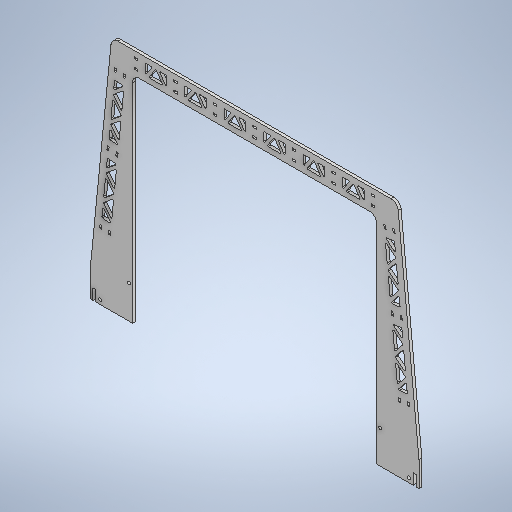
# Autodesk Inventor part: GateBrigeSideLessMaterial
Saved by Autodesk Inventor 2025.1 (Build 291241000, 241)
## iProperties
Created: 2025-03-30
Part Number: GateBrigeSideLessMaterial
Material: Všeobecné
Document SubType Name: Modeling
Designer: 42060
Density: 1 g/cm^3
Appearance: Výchozí
Author: 42060
Autodesk Inventor part; units mm, degrees
ref_plane "YZ Plane" through (0, 0, 0) normal (1, 0, 0) x (0, 1, 0)
ref_plane "XZ Plane" through (0, 0, 0) normal (0, 1, 0) x (-1, 0, 0)
ref_plane "XY Plane" through (0, 0, 0) normal (0, 0, 1) x (1, 0, 0)
sketch "Náčrt1" plane through (0, 0, 0) normal (0, 0, 1) x (1, 0, 0)
  line L0 (0, 0) -> (-160, 0)
  line L1 (-170, -10) -> (-170, -300)
  line L2 (-229, -300) -> (-229, -265.3)
  line L3 (-190.0509, 30) -> (0, 30)
  line L4 (0, 30) -> (0, 0)
  line L5 (-203.7, -249) -> (-170, -249)
  line L6 (-170, -249) -> (-170, -299)
  line L7 (-170, -299) -> (-220, -299)
  line L8 (-220, -299) -> (-220, -265.3)
  line L9 (-220, -265.3) -> (-203.7, -249)
  line L10 (-220, -299) -> (-170, -249) construction
  circle A0 centre (-215, -294) radius 2.1
  circle A1 centre (-175, -254) radius 2.1
  arc A2 (-160, 0) -> (-170, -10) centre (-160, -10) ccw
  line L11 (-200, 21.0077) -> (-229, -265.3)
  arc A3 (-190.0509, 30) -> (-200, 21.0077) centre (-190.0509, 20) ccw
  line L12 (-225, -300) -> (-225, -285)
  line L13 (-225, -285) -> (-221, -285)
  line L14 (-221, -285) -> (-221, -300)
  line L15 (-170, -300) -> (-221, -300)
  line L16 (-225, -300) -> (-229, -300)
  line L17 (0, 0) -> (160, 0)
  line L18 (170, -10) -> (170, -300)
  line L19 (229, -300) -> (229, -265.3)
  line L20 (190.0509, 30) -> (0, 30)
  line L21 (203.7, -249) -> (170, -249)
  line L22 (170, -249) -> (170, -299)
  line L23 (170, -299) -> (220, -299)
  line L24 (220, -299) -> (220, -265.3)
  line L25 (220, -265.3) -> (203.7, -249)
  line L26 (220, -299) -> (170, -249) construction
  circle A4 centre (215, -294) radius 2.1
  circle A5 centre (175, -254) radius 2.1
  arc A6 (170, -10) -> (160, 0) centre (160, -10) ccw
  line L27 (200, 21.0077) -> (229, -265.3)
  arc A7 (200, 21.0077) -> (190.0509, 30) centre (190.0509, 20) ccw
  line L28 (225, -300) -> (225, -285)
  line L29 (225, -285) -> (221, -285)
  line L30 (221, -285) -> (221, -300)
  line L31 (170, -300) -> (221, -300)
  line L32 (225, -300) -> (229, -300)
  line L33 (-36.6095, 9.0611) -> (-28.3278, 21.2788)
  line L34 (-26.6722, 21.2788) -> (-18.3905, 9.0611)
  line L35 (-19.2183, 7.5) -> (-35.7817, 7.5)
  line L36 (-21.6095, 20.9389) -> (-14.3278, 10.1964)
  line L37 (-12.5, 10.7575) -> (-12.5, 21.5)
  line L38 (-13.5, 22.5) -> (-20.7817, 22.5)
  line L39 (-33.3905, 20.9389) -> (-40.6722, 10.1964)
  line L40 (-42.5, 10.7575) -> (-42.5, 21.5)
  line L41 (-41.5, 22.5) -> (-34.2183, 22.5)
  line L42 (-55, 15) -> (0, 15) construction
  arc A8 (-41.5, 22.5) -> (-42.5, 21.5) centre (-41.5, 21.5) ccw
  arc A9 (-33.3905, 20.9389) -> (-34.2183, 22.5) centre (-34.2183, 21.5) ccw
  arc A10 (-42.5, 10.7575) -> (-40.6722, 10.1964) centre (-41.5, 10.7575) ccw
  arc A11 (-36.6095, 9.0611) -> (-35.7817, 7.5) centre (-35.7817, 8.5) ccw
  arc A12 (-19.2183, 7.5) -> (-18.3905, 9.0611) centre (-19.2183, 8.5) ccw
  arc A13 (-26.6722, 21.2788) -> (-28.3278, 21.2788) centre (-27.5, 20.7178) ccw
  arc A14 (-20.7817, 22.5) -> (-21.6095, 20.9389) centre (-20.7817, 21.5) ccw
  arc A15 (-12.5, 21.5) -> (-13.5, 22.5) centre (-13.5, 21.5) ccw
  arc A16 (-14.3278, 10.1964) -> (-12.5, 10.7575) centre (-13.5, 10.7575) ccw
  arc A17 (-81.6722, 21.2788) -> (-83.3278, 21.2788) centre (-82.5, 20.7178) ccw
  line L43 (-91.6095, 9.0611) -> (-83.3278, 21.2788)
  line L44 (-68.5, 22.5) -> (-75.7817, 22.5)
  arc A18 (-67.5, 21.5) -> (-68.5, 22.5) centre (-68.5, 21.5) ccw
  line L45 (-81.6722, 21.2788) -> (-73.3905, 9.0611)
  arc A19 (-74.2183, 7.5) -> (-73.3905, 9.0611) centre (-74.2183, 8.5) ccw
  line L46 (-76.6095, 20.9389) -> (-69.3278, 10.1964)
  line L47 (-74.2183, 7.5) -> (-90.7817, 7.5)
  arc A20 (-69.3278, 10.1964) -> (-67.5, 10.7575) centre (-68.5, 10.7575) ccw
  line L48 (-110, 15) -> (-55, 15) construction
  arc A21 (-96.5, 22.5) -> (-97.5, 21.5) centre (-96.5, 21.5) ccw
  arc A22 (-97.5, 10.7575) -> (-95.6722, 10.1964) centre (-96.5, 10.7575) ccw
  arc A23 (-91.6095, 9.0611) -> (-90.7817, 7.5) centre (-90.7817, 8.5) ccw
  arc A24 (-88.3905, 20.9389) -> (-89.2183, 22.5) centre (-89.2183, 21.5) ccw
  line L49 (-67.5, 10.7575) -> (-67.5, 21.5)
  arc A25 (-75.7817, 22.5) -> (-76.6095, 20.9389) centre (-75.7817, 21.5) ccw
  line L50 (-96.5, 22.5) -> (-89.2183, 22.5)
  line L51 (-88.3905, 20.9389) -> (-95.6722, 10.1964)
  line L52 (-97.5, 10.7575) -> (-97.5, 21.5)
  arc A26 (-136.6722, 21.2788) -> (-138.3278, 21.2788) centre (-137.5, 20.7178) ccw
  line L53 (-146.6095, 9.0611) -> (-138.3278, 21.2788)
  line L54 (-123.5, 22.5) -> (-130.7817, 22.5)
  arc A27 (-122.5, 21.5) -> (-123.5, 22.5) centre (-123.5, 21.5) ccw
  line L55 (-136.6722, 21.2788) -> (-128.3905, 9.0611)
  arc A28 (-129.2183, 7.5) -> (-128.3905, 9.0611) centre (-129.2183, 8.5) ccw
  line L56 (-131.6095, 20.9389) -> (-124.3278, 10.1964)
  line L57 (-129.2183, 7.5) -> (-145.7817, 7.5)
  arc A29 (-124.3278, 10.1964) -> (-122.5, 10.7575) centre (-123.5, 10.7575) ccw
  line L58 (-165, 15) -> (-110, 15) construction
  arc A30 (-151.5, 22.5) -> (-152.5, 21.5) centre (-151.5, 21.5) ccw
  arc A31 (-152.5, 10.7575) -> (-150.6722, 10.1964) centre (-151.5, 10.7575) ccw
  arc A32 (-146.6095, 9.0611) -> (-145.7817, 7.5) centre (-145.7817, 8.5) ccw
  arc A33 (-143.3905, 20.9389) -> (-144.2183, 22.5) centre (-144.2183, 21.5) ccw
  line L59 (-122.5, 10.7575) -> (-122.5, 21.5)
  arc A34 (-130.7817, 22.5) -> (-131.6095, 20.9389) centre (-130.7817, 21.5) ccw
  line L60 (-151.5, 22.5) -> (-144.2183, 22.5)
  line L61 (-143.3905, 20.9389) -> (-150.6722, 10.1964)
  line L62 (-152.5, 10.7575) -> (-152.5, 21.5)
  line L63 (-193.9606, -18.9513) -> (-184.0822, -19.9519)
  line L64 (-183.5507, -21.7216) -> (-194.4297, -30.5994)
  line L65 (-196.0568, -29.7239) -> (-195.0562, -19.8455)
  line L66 (-182.4936, -28.2252) -> (-184.6963, -49.9718)
  line L67 (-186.466, -50.5033) -> (-196.2379, -38.5286)
  line L68 (-196.0954, -37.1216) -> (-184.1208, -27.3497)
  line L69 (-195.9139, -45.2524) -> (-186.1419, -57.227)
  line L70 (-186.2844, -58.634) -> (-198.2591, -68.406)
  line L71 (-199.8862, -67.5304) -> (-197.6835, -45.7838)
  line L72 (-187.9502, -65.1562) -> (-199.9248, -74.9282)
  line L73 (-200.0673, -76.3352) -> (-190.2954, -88.3098)
  line L74 (-188.5257, -87.7783) -> (-186.323, -66.0318)
  line L75 (-199.7433, -83.0589) -> (-190.8655, -93.9379)
  line L76 (-191.741, -95.565) -> (-201.6194, -94.5645)
  line L77 (-202.5135, -93.4688) -> (-201.5129, -83.5904)
  line L78 (-189.0214, -19.4516) -> (-188.064, -10) construction
  arc A35 (-193.9606, -18.9513) -> (-195.0562, -19.8455) centre (-194.0613, -19.9463) ccw
  arc A36 (-183.5507, -21.7216) -> (-184.0822, -19.9519) centre (-184.1829, -20.9468) ccw
  arc A37 (-196.0568, -29.7239) -> (-194.4297, -30.5994) centre (-195.0619, -29.8246) ccw
  arc A38 (-196.0954, -37.1216) -> (-196.2379, -38.5286) centre (-195.4632, -37.8964) ccw
  arc A39 (-186.466, -50.5033) -> (-184.6963, -49.9718) centre (-185.6912, -49.871) ccw
  arc A40 (-182.4936, -28.2252) -> (-184.1208, -27.3497) centre (-183.4885, -28.1244) ccw
  arc A41 (-195.9139, -45.2524) -> (-197.6835, -45.7838) centre (-196.6886, -45.8846) ccw
  arc A42 (-186.2844, -58.634) -> (-186.1419, -57.227) centre (-186.9167, -57.8593) ccw
  arc A43 (-199.8862, -67.5304) -> (-198.2591, -68.406) centre (-198.8913, -67.6312) ccw
  arc A44 (-199.9248, -74.9282) -> (-200.0673, -76.3352) centre (-199.2926, -75.7029) ccw
  arc A45 (-190.2954, -88.3098) -> (-188.5257, -87.7783) centre (-189.5206, -87.6776) ccw
  arc A46 (-186.323, -66.0318) -> (-187.9502, -65.1562) centre (-187.3179, -65.931) ccw
  arc A47 (-199.7433, -83.0589) -> (-201.5129, -83.5904) centre (-200.518, -83.6912) ccw
  arc A48 (-202.5135, -93.4688) -> (-201.6194, -94.5645) centre (-201.5186, -93.5696) ccw
  arc A49 (-191.741, -95.565) -> (-190.8655, -93.9379) centre (-191.6402, -94.5701) ccw
  arc A50 (-212.5909, -192.9597) -> (-211.6968, -194.0554) centre (-211.596, -193.0605) ccw
  line L79 (-201.8184, -195.056) -> (-211.6968, -194.0554)
  arc A51 (-201.8184, -195.056) -> (-200.9429, -193.4288) centre (-201.7176, -194.0611) ccw
  arc A52 (-200.3728, -187.8008) -> (-198.6031, -187.2693) centre (-199.598, -187.1685) ccw
  line L80 (-209.8207, -182.5498) -> (-200.9429, -193.4288)
  line L81 (-212.5909, -192.9597) -> (-211.5903, -183.0813)
  arc A53 (-209.8207, -182.5498) -> (-211.5903, -183.0813) centre (-210.5954, -183.1821) ccw
  line L82 (-198.0276, -164.6471) -> (-210.0022, -174.4191)
  line L83 (-210.1447, -175.8261) -> (-200.3728, -187.8008)
  line L84 (-198.6031, -187.2693) -> (-196.4004, -165.5227)
  arc A54 (-210.0022, -174.4191) -> (-210.1447, -175.8261) centre (-209.37, -175.1939) ccw
  arc A55 (-209.9636, -167.0214) -> (-208.3365, -167.8969) centre (-208.9687, -167.1221) ccw
  arc A56 (-196.4004, -165.5227) -> (-198.0276, -164.6471) centre (-197.3953, -165.4219) ccw
  line L85 (-205.9913, -144.7433) -> (-196.2193, -156.7179)
  arc A57 (-196.3618, -158.125) -> (-196.2193, -156.7179) centre (-196.9941, -157.3502) ccw
  line L86 (-209.9636, -167.0214) -> (-207.7609, -145.2748)
  line L87 (-196.3618, -158.125) -> (-208.3365, -167.8969)
  arc A58 (-196.5434, -149.9942) -> (-194.7737, -149.4627) centre (-195.7686, -149.362) ccw
  arc A59 (-205.9913, -144.7433) -> (-207.7609, -145.2748) centre (-206.766, -145.3755) ccw
  line L88 (-196.5434, -149.9942) -> (-206.3153, -138.0196)
  arc A60 (-206.1728, -136.6125) -> (-206.3153, -138.0196) centre (-205.5406, -137.3873) ccw
  arc A61 (-206.1342, -129.2148) -> (-204.5071, -130.0903) centre (-205.1393, -129.3156) ccw
  line L89 (-192.571, -127.7161) -> (-194.7737, -149.4627)
  line L90 (-206.1728, -136.6125) -> (-194.1982, -126.8406)
  arc A62 (-192.571, -127.7161) -> (-194.1982, -126.8406) centre (-193.5659, -127.6154) ccw
  arc A63 (-193.6281, -121.2125) -> (-194.1596, -119.4429) centre (-194.2603, -120.4378) ccw
  line L91 (-199.0988, -118.9426) -> (-198.1414, -109.4909) construction
  line L92 (-204.038, -118.4423) -> (-194.1596, -119.4429)
  arc A64 (-204.038, -118.4423) -> (-205.1336, -119.3364) centre (-204.1387, -119.4372) ccw
  line L93 (-193.6281, -121.2125) -> (-204.5071, -130.0903)
  line L94 (-206.1342, -129.2148) -> (-205.1336, -119.3364)
  line L95 (36.6095, 9.0611) -> (28.3278, 21.2788)
  line L96 (26.6722, 21.2788) -> (18.3905, 9.0611)
  line L97 (19.2183, 7.5) -> (35.7817, 7.5)
  line L98 (21.6095, 20.9389) -> (14.3278, 10.1964)
  line L99 (12.5, 10.7575) -> (12.5, 21.5)
  line L100 (13.5, 22.5) -> (20.7817, 22.5)
  line L101 (33.3905, 20.9389) -> (40.6722, 10.1964)
  line L102 (42.5, 10.7575) -> (42.5, 21.5)
  line L103 (41.5, 22.5) -> (34.2183, 22.5)
  line L104 (55, 15) -> (0, 15) construction
  arc A65 (42.5, 21.5) -> (41.5, 22.5) centre (41.5, 21.5) ccw
  arc A66 (34.2183, 22.5) -> (33.3905, 20.9389) centre (34.2183, 21.5) ccw
  arc A67 (40.6722, 10.1964) -> (42.5, 10.7575) centre (41.5, 10.7575) ccw
  arc A68 (35.7817, 7.5) -> (36.6095, 9.0611) centre (35.7817, 8.5) ccw
  arc A69 (18.3905, 9.0611) -> (19.2183, 7.5) centre (19.2183, 8.5) ccw
  arc A70 (28.3278, 21.2788) -> (26.6722, 21.2788) centre (27.5, 20.7178) ccw
  arc A71 (21.6095, 20.9389) -> (20.7817, 22.5) centre (20.7817, 21.5) ccw
  arc A72 (13.5, 22.5) -> (12.5, 21.5) centre (13.5, 21.5) ccw
  arc A73 (12.5, 10.7575) -> (14.3278, 10.1964) centre (13.5, 10.7575) ccw
  line L105 (67.5, 10.7575) -> (67.5, 21.5)
  line L106 (96.5, 22.5) -> (89.2183, 22.5)
  arc A74 (97.5, 21.5) -> (96.5, 22.5) centre (96.5, 21.5) ccw
  line L107 (97.5, 10.7575) -> (97.5, 21.5)
  arc A75 (95.6722, 10.1964) -> (97.5, 10.7575) centre (96.5, 10.7575) ccw
  arc A76 (67.5, 10.7575) -> (69.3278, 10.1964) centre (68.5, 10.7575) ccw
  arc A77 (68.5, 22.5) -> (67.5, 21.5) centre (68.5, 21.5) ccw
  arc A78 (89.2183, 22.5) -> (88.3905, 20.9389) centre (89.2183, 21.5) ccw
  arc A79 (83.3278, 21.2788) -> (81.6722, 21.2788) centre (82.5, 20.7178) ccw
  line L108 (88.3905, 20.9389) -> (95.6722, 10.1964)
  line L109 (91.6095, 9.0611) -> (83.3278, 21.2788)
  arc A80 (76.6095, 20.9389) -> (75.7817, 22.5) centre (75.7817, 21.5) ccw
  arc A81 (90.7817, 7.5) -> (91.6095, 9.0611) centre (90.7817, 8.5) ccw
  line L110 (110, 15) -> (55, 15) construction
  line L111 (68.5, 22.5) -> (75.7817, 22.5)
  line L112 (76.6095, 20.9389) -> (69.3278, 10.1964)
  line L113 (81.6722, 21.2788) -> (73.3905, 9.0611)
  arc A82 (73.3905, 9.0611) -> (74.2183, 7.5) centre (74.2183, 8.5) ccw
  line L114 (74.2183, 7.5) -> (90.7817, 7.5)
  line L115 (122.5, 10.7575) -> (122.5, 21.5)
  line L116 (151.5, 22.5) -> (144.2183, 22.5)
  arc A83 (152.5, 21.5) -> (151.5, 22.5) centre (151.5, 21.5) ccw
  line L117 (152.5, 10.7575) -> (152.5, 21.5)
  arc A84 (150.6722, 10.1964) -> (152.5, 10.7575) centre (151.5, 10.7575) ccw
  arc A85 (122.5, 10.7575) -> (124.3278, 10.1964) centre (123.5, 10.7575) ccw
  arc A86 (123.5, 22.5) -> (122.5, 21.5) centre (123.5, 21.5) ccw
  arc A87 (144.2183, 22.5) -> (143.3905, 20.9389) centre (144.2183, 21.5) ccw
  arc A88 (138.3278, 21.2788) -> (136.6722, 21.2788) centre (137.5, 20.7178) ccw
  line L118 (143.3905, 20.9389) -> (150.6722, 10.1964)
  line L119 (146.6095, 9.0611) -> (138.3278, 21.2788)
  arc A89 (131.6095, 20.9389) -> (130.7817, 22.5) centre (130.7817, 21.5) ccw
  arc A90 (145.7817, 7.5) -> (146.6095, 9.0611) centre (145.7817, 8.5) ccw
  line L120 (165, 15) -> (110, 15) construction
  line L121 (123.5, 22.5) -> (130.7817, 22.5)
  line L122 (131.6095, 20.9389) -> (124.3278, 10.1964)
  line L123 (136.6722, 21.2788) -> (128.3905, 9.0611)
  arc A91 (128.3905, 9.0611) -> (129.2183, 7.5) centre (129.2183, 8.5) ccw
  line L124 (129.2183, 7.5) -> (145.7817, 7.5)
  line L125 (193.9606, -18.9513) -> (184.0822, -19.9519)
  line L126 (183.5507, -21.7216) -> (194.4297, -30.5994)
  line L127 (196.0568, -29.7239) -> (195.0562, -19.8455)
  line L128 (182.4936, -28.2252) -> (184.6963, -49.9718)
  line L129 (186.466, -50.5033) -> (196.2379, -38.5286)
  line L130 (196.0954, -37.1216) -> (184.1208, -27.3497)
  line L131 (195.9139, -45.2524) -> (186.1419, -57.227)
  line L132 (186.2844, -58.634) -> (198.2591, -68.406)
  line L133 (199.8862, -67.5304) -> (197.6835, -45.7838)
  line L134 (187.9502, -65.1562) -> (199.9248, -74.9282)
  line L135 (200.0673, -76.3352) -> (190.2954, -88.3098)
  line L136 (188.5257, -87.7783) -> (186.323, -66.0318)
  line L137 (199.7433, -83.0589) -> (190.8655, -93.9379)
  line L138 (191.741, -95.565) -> (201.6194, -94.5645)
  line L139 (202.5135, -93.4688) -> (201.5129, -83.5904)
  arc A92 (195.0562, -19.8455) -> (193.9606, -18.9513) centre (194.0613, -19.9463) ccw
  arc A93 (184.0822, -19.9519) -> (183.5507, -21.7216) centre (184.1829, -20.9468) ccw
  arc A94 (194.4297, -30.5994) -> (196.0568, -29.7239) centre (195.0619, -29.8246) ccw
  arc A95 (196.2379, -38.5286) -> (196.0954, -37.1216) centre (195.4632, -37.8964) ccw
  arc A96 (184.6963, -49.9718) -> (186.466, -50.5033) centre (185.6912, -49.871) ccw
  arc A97 (184.1208, -27.3497) -> (182.4936, -28.2252) centre (183.4885, -28.1244) ccw
  arc A98 (197.6835, -45.7838) -> (195.9139, -45.2524) centre (196.6886, -45.8846) ccw
  arc A99 (186.1419, -57.227) -> (186.2844, -58.634) centre (186.9167, -57.8593) ccw
  arc A100 (198.2591, -68.406) -> (199.8862, -67.5304) centre (198.8913, -67.6312) ccw
  arc A101 (200.0673, -76.3352) -> (199.9248, -74.9282) centre (199.2926, -75.7029) ccw
  arc A102 (188.5257, -87.7783) -> (190.2954, -88.3098) centre (189.5206, -87.6776) ccw
  arc A103 (187.9502, -65.1562) -> (186.323, -66.0318) centre (187.3179, -65.931) ccw
  arc A104 (201.5129, -83.5904) -> (199.7433, -83.0589) centre (200.518, -83.6912) ccw
  arc A105 (201.6194, -94.5645) -> (202.5135, -93.4688) centre (201.5186, -93.5696) ccw
  arc A106 (190.8655, -93.9379) -> (191.741, -95.565) centre (191.6402, -94.5701) ccw
  arc A107 (194.1596, -119.4429) -> (193.6281, -121.2125) centre (194.2603, -120.4378) ccw
  arc A108 (194.1982, -126.8406) -> (192.571, -127.7161) centre (193.5659, -127.6154) ccw
  line L140 (204.038, -118.4423) -> (194.1596, -119.4429)
  line L141 (193.6281, -121.2125) -> (204.5071, -130.0903)
  line L142 (206.1342, -129.2148) -> (205.1336, -119.3364)
  line L143 (206.1728, -136.6125) -> (194.1982, -126.8406)
  arc A109 (205.1336, -119.3364) -> (204.038, -118.4423) centre (204.1387, -119.4372) ccw
  arc A110 (204.5071, -130.0903) -> (206.1342, -129.2148) centre (205.1393, -129.3156) ccw
  line L144 (192.571, -127.7161) -> (194.7737, -149.4627)
  arc A111 (207.7609, -145.2748) -> (205.9913, -144.7433) centre (206.766, -145.3755) ccw
  line L145 (196.5434, -149.9942) -> (206.3153, -138.0196)
  arc A112 (206.3153, -138.0196) -> (206.1728, -136.6125) centre (205.5406, -137.3873) ccw
  arc A113 (194.7737, -149.4627) -> (196.5434, -149.9942) centre (195.7686, -149.362) ccw
  line L146 (205.9913, -144.7433) -> (196.2193, -156.7179)
  arc A114 (196.2193, -156.7179) -> (196.3618, -158.125) centre (196.9941, -157.3502) ccw
  arc A115 (198.0276, -164.6471) -> (196.4004, -165.5227) centre (197.3953, -165.4219) ccw
  line L147 (196.3618, -158.125) -> (208.3365, -167.8969)
  arc A116 (208.3365, -167.8969) -> (209.9636, -167.0214) centre (208.9687, -167.1221) ccw
  line L148 (209.9636, -167.0214) -> (207.7609, -145.2748)
  arc A117 (200.9429, -193.4288) -> (201.8184, -195.056) centre (201.7176, -194.0611) ccw
  arc A118 (211.6968, -194.0554) -> (212.5909, -192.9597) centre (211.596, -193.0605) ccw
  arc A119 (198.6031, -187.2693) -> (200.3728, -187.8008) centre (199.598, -187.1685) ccw
  line L149 (212.5909, -192.9597) -> (211.5903, -183.0813)
  line L150 (209.8207, -182.5498) -> (200.9429, -193.4288)
  arc A120 (211.5903, -183.0813) -> (209.8207, -182.5498) centre (210.5954, -183.1821) ccw
  line L151 (210.1447, -175.8261) -> (200.3728, -187.8008)
  arc A121 (210.1447, -175.8261) -> (210.0022, -174.4191) centre (209.37, -175.1939) ccw
  line L152 (198.6031, -187.2693) -> (196.4004, -165.5227)
  line L153 (198.0276, -164.6471) -> (210.0022, -174.4191)
  line L154 (201.8184, -195.056) -> (211.6968, -194.0554)
  line L155 (-2.5, 10) -> (2.5, 10)
  line L156 (2.5, 10) -> (2.5, 7.5)
  line L157 (2.5, 7.5) -> (-2.5, 7.5)
  line L158 (-2.5, 7.5) -> (-2.5, 10)
  line L159 (-2.5, 22.5) -> (2.5, 22.5)
  line L160 (2.5, 22.5) -> (2.5, 20)
  line L161 (2.5, 20) -> (-2.5, 20)
  line L162 (-2.5, 20) -> (-2.5, 22.5)
  line L163 (0, 20) -> (0, 10) construction
  line L164 (-42.5, 10.7575) -> (-42.5, 7.5) construction
  line L165 (-42.5, 7.5) -> (-40.6722, 10.1964) construction
  line L166 (-27.5, 22.5) -> (-27.5, 7.5) construction
  line L167 (-52.5, 10) -> (-52.5, 7.5)
  line L168 (-57.5, 10) -> (-52.5, 10)
  line L169 (-52.5, 7.5) -> (-57.5, 7.5)
  line L170 (-57.5, 7.5) -> (-57.5, 10)
  line L171 (-57.5, 22.5) -> (-52.5, 22.5)
  line L172 (-52.5, 20) -> (-57.5, 20)
  line L173 (-57.5, 20) -> (-57.5, 22.5)
  line L174 (-52.5, 22.5) -> (-52.5, 20)
  line L175 (-107.5, 10) -> (-107.5, 7.5)
  line L176 (-112.5, 10) -> (-107.5, 10)
  line L177 (-107.5, 7.5) -> (-112.5, 7.5)
  line L178 (-112.5, 7.5) -> (-112.5, 10)
  line L179 (-112.5, 22.5) -> (-107.5, 22.5)
  line L180 (-107.5, 20) -> (-112.5, 20)
  line L181 (-112.5, 20) -> (-112.5, 22.5)
  line L182 (-107.5, 22.5) -> (-107.5, 20)
  line L183 (-162.5, 10) -> (-162.5, 7.5)
  line L184 (-167.5, 10) -> (-162.5, 10)
  line L185 (-162.5, 7.5) -> (-167.5, 7.5)
  line L186 (-167.5, 7.5) -> (-167.5, 10)
  line L187 (-167.5, 22.5) -> (-162.5, 22.5)
  line L188 (-162.5, 20) -> (-167.5, 20)
  line L189 (-167.5, 20) -> (-167.5, 22.5)
  line L190 (-162.5, 22.5) -> (-162.5, 20)
  line L191 (52.5, 20) -> (52.5, 22.5)
  line L192 (57.5, 20) -> (52.5, 20)
  line L193 (57.5, 22.5) -> (57.5, 20)
  line L194 (52.5, 22.5) -> (57.5, 22.5)
  line L195 (57.5, 10) -> (57.5, 7.5)
  line L196 (52.5, 10) -> (57.5, 10)
  line L197 (57.5, 7.5) -> (52.5, 7.5)
  line L198 (52.5, 7.5) -> (52.5, 10)
  line L199 (107.5, 20) -> (107.5, 22.5)
  line L200 (112.5, 20) -> (107.5, 20)
  line L201 (112.5, 22.5) -> (112.5, 20)
  line L202 (107.5, 22.5) -> (112.5, 22.5)
  line L203 (112.5, 10) -> (112.5, 7.5)
  line L204 (107.5, 10) -> (112.5, 10)
  line L205 (112.5, 7.5) -> (107.5, 7.5)
  line L206 (107.5, 7.5) -> (107.5, 10)
  line L207 (162.5, 20) -> (162.5, 22.5)
  line L208 (167.5, 20) -> (162.5, 20)
  line L209 (167.5, 22.5) -> (167.5, 20)
  line L210 (162.5, 22.5) -> (167.5, 22.5)
  line L211 (167.5, 10) -> (167.5, 7.5)
  line L212 (162.5, 10) -> (167.5, 10)
  line L213 (167.5, 7.5) -> (162.5, 7.5)
  line L214 (162.5, 7.5) -> (162.5, 10)
  line L215 (-195.022, -4.2696) -> (-192.5347, -4.5216)
  line L216 (-192.5347, -4.5216) -> (-193.0386, -9.4961)
  line L217 (-193.0386, -9.4961) -> (-195.5258, -9.2442)
  line L218 (-195.5258, -9.2442) -> (-195.022, -4.2696)
  line L219 (-182.5856, -5.5293) -> (-180.0983, -5.7813)
  line L220 (-180.0983, -5.7813) -> (-180.6022, -10.7558)
  line L221 (-180.6022, -10.7558) -> (-183.0895, -10.5039)
  line L222 (-183.0895, -10.5039) -> (-182.5856, -5.5293)
  line L223 (-193.0386, -9.4961) -> (-183.0895, -10.5039) construction
  line L224 (-205.6032, -108.7351) -> (-205.0994, -103.7606)
  line L225 (-202.6121, -104.0125) -> (-203.116, -108.9871)
  line L226 (-203.116, -108.9871) -> (-205.6032, -108.7351)
  line L227 (-205.0994, -103.7606) -> (-202.6121, -104.0125)
  line L228 (-193.1669, -109.9948) -> (-192.663, -105.0203)
  line L229 (-190.6796, -110.2467) -> (-193.1669, -109.9948)
  line L230 (-190.1757, -105.2722) -> (-190.6796, -110.2467)
  line L231 (-192.663, -105.0203) -> (-190.1757, -105.2722)
  line L232 (-203.116, -108.9871) -> (-193.1669, -109.9948) construction
  line L233 (-202.6121, -104.0125) -> (-192.663, -105.0203) construction
  line L234 (-197.6375, -104.5164) -> (-196.6802, -95.0647) construction
  line L235 (-215.6806, -208.2261) -> (-215.1768, -203.2515)
  line L236 (-212.6895, -203.5035) -> (-213.1934, -208.478)
  line L237 (-213.1934, -208.478) -> (-215.6806, -208.2261)
  line L238 (-215.1768, -203.2515) -> (-212.6895, -203.5035)
  line L239 (-203.2443, -209.4857) -> (-202.7404, -204.5112)
  line L240 (-200.757, -209.7377) -> (-203.2443, -209.4857)
  line L241 (-200.2531, -204.7631) -> (-200.757, -209.7377)
  line L242 (-202.7404, -204.5112) -> (-200.2531, -204.7631)
  line L243 (-213.1934, -208.478) -> (-203.2443, -209.4857) construction
  line L244 (195.022, -4.2696) -> (192.5347, -4.5216)
  line L245 (192.5347, -4.5216) -> (193.0386, -9.4961)
  line L246 (193.0386, -9.4961) -> (195.5258, -9.2442)
  line L247 (195.5258, -9.2442) -> (195.022, -4.2696)
  line L248 (182.5856, -5.5293) -> (180.0983, -5.7813)
  line L249 (180.0983, -5.7813) -> (180.6022, -10.7558)
  line L250 (180.6022, -10.7558) -> (183.0895, -10.5039)
  line L251 (183.0895, -10.5039) -> (182.5856, -5.5293)
  line L252 (205.6032, -108.7351) -> (205.0994, -103.7606)
  line L253 (202.6121, -104.0125) -> (203.116, -108.9871)
  line L254 (203.116, -108.9871) -> (205.6032, -108.7351)
  line L255 (205.0994, -103.7606) -> (202.6121, -104.0125)
  line L256 (193.1669, -109.9948) -> (192.663, -105.0203)
  line L257 (190.6796, -110.2467) -> (193.1669, -109.9948)
  line L258 (190.1757, -105.2722) -> (190.6796, -110.2467)
  line L259 (192.663, -105.0203) -> (190.1757, -105.2722)
  line L260 (215.6806, -208.2261) -> (215.1768, -203.2515)
  line L261 (212.6895, -203.5035) -> (213.1934, -208.478)
  line L262 (213.1934, -208.478) -> (215.6806, -208.2261)
  line L263 (215.1768, -203.2515) -> (212.6895, -203.5035)
  line L264 (203.2443, -209.4857) -> (202.7404, -204.5112)
  line L265 (200.757, -209.7377) -> (203.2443, -209.4857)
  line L266 (200.2531, -204.7631) -> (200.757, -209.7377)
  line L267 (202.7404, -204.5112) -> (200.2531, -204.7631)
  point P0 (-12.5, 7.5)
  point P1 (-32.3323, 22.5)
  point P2 (-42.5, 22.5)
  point P3 (-27.5, 15)
  point P4 (-12.5, 16.1288)
  point P5 (-82.5, 22.5)
  point P6 (-82.5, 15)
  point P7 (-82.5, 7.5)
  point P8 (-87.3323, 22.5)
  point P9 (-97.5, 22.5)
  point P10 (-67.5, 7.5)
  point P11 (-67.5, 16.1288)
  point P12 (-137.5, 22.5)
  point P13 (-137.5, 15)
  point P14 (-137.5, 7.5)
  point P15 (-142.3323, 22.5)
  point P16 (-152.5, 22.5)
  point P17 (-122.5, 7.5)
  point P18 (-122.5, 16.1288)
  point P19 (-194.9555, -18.8506)
  point P20 (-181.6802, -20.1952)
  point P21 (-196.3001, -32.1258)
  point P22 (-182.2503, -25.8233)
  point P23 (-184.9396, -52.3737)
  point P24 (-196.8702, -37.7539)
  point P25 (-197.4402, -43.3819)
  point P26 (-185.5097, -58.0018)
  point P27 (-200.1295, -69.9324)
  point P28 (-186.0797, -63.6298)
  point P29 (-200.6996, -75.5604)
  point P30 (-188.769, -90.1803)
  point P31 (-201.2696, -81.1885)
  point P32 (-189.3391, -95.8083)
  point P33 (-202.6143, -94.4637)
  point P34 (-212.6917, -193.9546)
  point P35 (-199.4165, -195.2993)
  point P36 (-198.8464, -189.6712)
  point P37 (-211.347, -180.6794)
  point P38 (-210.777, -175.0513)
  point P39 (-210.2069, -169.4233)
  point P40 (-196.1571, -163.1208)
  point P41 (-195.5871, -157.4927)
  point P42 (-195.017, -151.8647)
  point P43 (-207.5176, -142.8728)
  point P44 (-206.9476, -137.2448)
  point P45 (-206.3775, -131.6167)
  point P46 (-192.3277, -125.3142)
  point P47 (-191.7576, -119.6862)
  point P48 (-205.0329, -118.3415)
  point P49 (27.5, 22.5)
  point P50 (12.5, 7.5)
  point P51 (32.3323, 22.5)
  point P52 (42.5, 22.5)
  point P53 (27.5, 7.5)
  point P54 (27.5, 15)
  point P55 (12.5, 16.1288)
  point P56 (67.5, 7.5)
  point P57 (67.5, 16.1288)
  point P58 (82.5, 22.5)
  point P59 (87.3323, 22.5)
  point P60 (97.5, 22.5)
  point P61 (82.5, 15)
  point P62 (82.5, 7.5)
  point P63 (122.5, 7.5)
  point P64 (122.5, 16.1288)
  point P65 (137.5, 22.5)
  point P66 (142.3323, 22.5)
  point P67 (152.5, 22.5)
  point P68 (137.5, 15)
  point P69 (137.5, 7.5)
  point P70 (194.9555, -18.8506)
  point P71 (181.6802, -20.1952)
  point P72 (196.3001, -32.1258)
  point P73 (182.2503, -25.8233)
  point P74 (184.9396, -52.3737)
  point P75 (196.8702, -37.7539)
  point P76 (197.4402, -43.3819)
  point P77 (185.5097, -58.0018)
  point P78 (200.1295, -69.9324)
  point P79 (186.0797, -63.6298)
  point P80 (200.6996, -75.5604)
  point P81 (188.769, -90.1803)
  point P82 (201.2696, -81.1885)
  point P83 (189.3391, -95.8083)
  point P84 (202.6143, -94.4637)
  point P85 (189.0214, -19.4516)
  point P86 (191.7576, -119.6862)
  point P87 (192.3277, -125.3142)
  point P88 (199.0988, -118.9426)
  point P89 (205.0329, -118.3415)
  point P90 (206.3775, -131.6167)
  point P91 (206.9476, -137.2448)
  point P92 (195.017, -151.8647)
  point P93 (207.5176, -142.8728)
  point P94 (195.5871, -157.4927)
  point P95 (196.1571, -163.1208)
  point P96 (210.2069, -169.4233)
  point P97 (212.6917, -193.9546)
  point P98 (199.4165, -195.2993)
  point P99 (198.8464, -189.6712)
  point P100 (210.777, -175.0513)
  point P101 (211.347, -180.6794)
  point P102 (0, 15)
  point P103 (-27.5, 15)
  point P104 (-55, 10)
  point P105 (-55, 20)
  point P106 (-110, 10)
  point P107 (-110, 20)
  point P108 (-165, 10)
  point P109 (-165, 20)
  point P110 (55, 20)
  point P111 (55, 10)
  point P112 (110, 20)
  point P113 (110, 10)
  point P114 (165, 20)
  point P115 (165, 10)
  point P116 (-208.2188, -208.9819)
  dimension "d0" = 50
  dimension "d1" = 50
  dimension "d3" = 33.7
  dimension "d4" = 45
  dimension "d5" = 0
  dimension "d6" = 4.2
  dimension "d7" = 5
  dimension "d8" = 5
  dimension "d10" = 170
  dimension "d12" = 30
  dimension "d14" = 10
  dimension "d16" = 15
  dimension "d17" = 1
  dimension "d18" = 4
  dimension "d19" = 1
  dimension "d20" = 4
  dimension "d21" = 300
  dimension "d22" = 30
  dimension "d46" = 4
  dimension "d47" = 4
  dimension "d50" = 15
  dimension "d51" = 30
  dimension "d52" = 1
  dimension "d55" = 55
  dimension "d63" = 4
  dimension "d64" = 4
  dimension "d65" = 4
  dimension "d66" = 4
  dimension "d67" = 1
  dimension "d70" = 100
  dimension "d77" = 55
  dimension "d84" = 100
  dimension "d91" = 2.5
  dimension "d92" = 5
  dimension "d93" = 15
  dimension "d96" = 55
  dimension "d103" = 55
  dimension "d108" = 5
  dimension "d109" = 2.5
  dimension "d110" = 7.5
  dimension "d111" = 15
  dimension "d115" = 100
  dimension "d122" = 9.5
  constraints: 536 end point, 236 point on circle, 226 point on line, 141 symmetric about line, 122 centre point, 52 tangent, 24 equal radius, 23 perpendicular, 20 parallel, 12 midpoint, 11 collinear, 10 coincident, 10 horizontal, 6 equal length, 4 horizontal alignment, 4 vertical alignment, 2 vertical, 579 other
  measures "d0" distance of L5.end L6.end
  measures "d1" distance of L6.end L7.end
  measures "d3" distance of L5.start L5.end
  measures "d4" angle of L5 L9
  measures "d5" distance between parallel lines of L1 L6
  measures "d6" diameter of A1
  measures "d7" distance from line of L5 A1.centre
  measures "d8" distance from line of L7 A0.centre
  measures "d10" distance between parallel lines of L1 L4
  measures "d12" distance between parallel lines of L0 L3
  measures "d14" radius of A3
  measures "d16" distance between parallel lines of L16 L13
  measures "d17" distance between parallel lines of L7 L15
  measures "d18" distance between parallel lines of L14 L12
  measures "d19" distance between parallel lines of L8 L14
  measures "d20" distance between parallel lines of L12 L2
  measures "d21" distance between parallel lines of L15 L0
  measures "d22" distance from line of L11.start L1
  measures "d46" distance between parallel lines of L33 L39
  measures "d47" distance between parallel lines of L36 L34
  measures "d50" distance from line of L35 L166.start
  measures "d51" distance between parallel lines of L37 L40
  measures "d52" radius of A8
  measures "d55" distance of L166.start point (-82.5, 22.5)
  measures "d63" distance between parallel lines of L68 L64
  measures "d64" distance between parallel lines of L69 L67
  measures "d65" distance between parallel lines of L72 L70
  measures "d66" distance between parallel lines of L73 L75
  measures "d67" radius of A35
  measures "d70" distance of point (-202.614, -94.464) point (-212.692, -193.955)
  measures "d77" distance of point (12.5, 7.5) point (67.5, 7.5)
  measures "d84" distance of point (181.68, -20.195) point (191.758, -119.686)
  measures "d91" distance of L159.end L160.end
  measures "d92" distance of L159.start L159.end
  measures "d93" distance between parallel lines of L157 L159
  measures "d96" distance of L155.end L167.start
  measures "d103" distance of L159.start L191.end
  measures "d108" distance of L217.end L215.start
  measures "d109" distance of L215.start L215.end
  measures "d110" distance between parallel lines of L11 L218
  measures "d111" distance between parallel lines of L220 L218
  measures "d115" distance of L217.end L224.start
  measures "d122" distance of L78.start L78.end
extrude "Vysunutí1" add sketch "Náčrt1" along normal blind 4 contours L0 A2 L1 L5 L9 L8 L7 L15 L14 L13 L12 L16 L2 L11 A3 L3 L4 L159 L162 L161 L155 L158 L157 | L4 L157 L156 L155 L161 L160 L159 L20 A7 L27 L19 L32 L28 L29 L30 L31 L18 L23 L24 L25 L21 A6 L17 | L1 L7 L8 L9 L5 | L21 L25 L24 L23 L18
equation "\"d44\" = d18"
